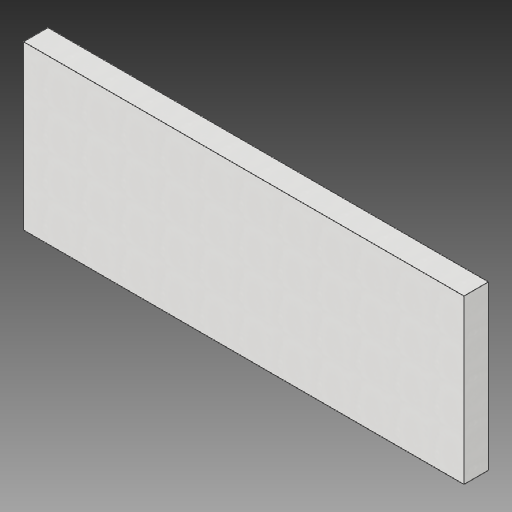
# Autodesk Inventor part: Перекрытие коридора
Saved by Autodesk Inventor 2019 (Build 230136000, 136)
## iProperties
Created: 2018-10-10
Part Number: Перекрытие коридора
Material: Гипсокартон
Document SubType Name: Modeling
Designer: Андреев Н.Л.
Density: 1.1 g/cm^3
Appearance: Гипсокартон — окрашенный — белый
Author: Андреев Н.Л.
Autodesk Inventor part; units mm, degrees
ref_plane "YZ Plane" through (0, 0, 0) normal (1, 0, 0) x (0, 1, 0)
ref_plane "XZ Plane" through (0, 0, 0) normal (0, 1, 0) x (-1, 0, 0)
ref_plane "XY Plane" through (0, 0, 0) normal (0, 0, 1) x (1, 0, 0)
sketch "Эскиз1" plane through (0, 0, 0) normal (0, 0, 1) x (1, 0, 0)
  line L0 (-1500, 2600) -> (-1500, -1200) construction
  line L1 (-1500, -1200) -> (-9900, -1200) construction
  line L2 (-9900, -1200) -> (-9900, 2600) construction
  line L3 (-9900, 2600) -> (-1500, 2600) construction
  line L4 (-1500, 3000) -> (-9900, 3000) construction
  line L5 (-9900, 3000) -> (-9900, 5000) construction
  line L6 (-9900, 5000) -> (-7000, 5000) construction
  line L7 (-7000, 5000) -> (-7000, 5400) construction
  line L8 (-7000, 5400) -> (-9900, 5400) construction
  line L9 (-9900, 5400) -> (-9900, 9200) construction
  line L10 (-9900, 9200) -> (-1500, 9200) construction
  line L11 (-1500, 9200) -> (-1500, 3000) construction
  line L12 (-10300, -200) -> (-10300, -1600) construction
  line L13 (-10300, -1600) -> (-1100, -1600) construction
  line L14 (-1100, -1600) -> (-1100, -200) construction
  line L15 (-1100, -200) -> (1100, -200) construction
  line L16 (1100, -200) -> (1100, -600) construction
  line L17 (1100, -600) -> (7500, -600) construction
  line L18 (7500, -600) -> (7500, 8600) construction
  line L19 (7500, 8600) -> (1100, 8600) construction
  line L20 (1100, 8600) -> (1100, 8200) construction
  line L21 (1100, 8200) -> (-1100, 8200) construction
  line L22 (-1100, 8200) -> (-1100, 9600) construction
  line L23 (-1100, 9600) -> (-10300, 9600) construction
  line L24 (-10300, 9600) -> (-10300, 8600) construction
  line L25 (-10300, 8600) -> (-18900, 8600) construction
  line L26 (-18900, 8600) -> (-18900, -600) construction
  line L27 (-18900, -600) -> (-12500, -600) construction
  line L28 (-12500, -600) -> (-12500, -200) construction
  line L29 (-12500, -200) -> (-10300, -200) construction
  line L30 (-1100, 7800) -> (1100, 7800) construction
  line L31 (1100, 7800) -> (1100, 200) construction
  line L32 (1100, 200) -> (-1100, 200) construction
  line L33 (-1100, 200) -> (-1100, 7800) construction
  line L34 (-18500, -200) -> (-18500, 8200) construction
  line L35 (-18500, 8200) -> (-12900, 8200) construction
  line L36 (-12900, 8200) -> (-12900, -200) construction
  line L37 (-12900, -200) -> (-18500, -200) construction
  line L38 (1500, -200) -> (1500, 8200) construction
  line L39 (1500, 8200) -> (7100, 8200) construction
  line L40 (7100, 8200) -> (7100, -200) construction
  line L41 (7100, -200) -> (1500, -200) construction
  line L42 (-10300, 200) -> (-12500, 200) construction
  line L43 (-12500, 200) -> (-12500, 8200) construction
  line L44 (-12500, 8200) -> (-10300, 8200) construction
  line L45 (-10300, 8200) -> (-10300, 200) construction
  line L46 (-6900, 3000) -> (-1500, 3000)
  line L47 (-1500, 3000) -> (-1500, 5000)
  line L48 (-1500, 5000) -> (-6900, 5000)
  line L49 (-6900, 5000) -> (-6900, 3000)
  point P0 (0, 0)
  dimension "d0" = 3000
  constraints: 8 end point, 2 parallel, 2 point on line, 1 collinear, 1 horizontal, 1 perpendicular
  measures "d0" distance between parallel lines of L49 L5
extrude "Выдавливание1" add sketch "Эскиз1" against normal blind 300
equation "\"d0\" = зДл"
equation "\"d1\" = зТолПерекрытия"
equation "\"зДл\" = 3000"
equation "\"пПодъем\" = 162.5"
equation "\"пХод\" = 296.8"
equation "\"пЭффШаг\" = 621.8"
equation "\"пСвес\" = 30.2"
equation "\"пОтступСтен\" = 5"
equation "\"пДиаг\" = 338.3733"
equation "\"пШирПроступи\" = 327"
equation "\"пТолПодступенка\" = 17.4"
equation "\"пГлубПаза\" = 12"
equation "\"пОтступОтСтен\" = 5"
equation "\"пТолПричала\" = 17.4"
equation "\"зТолПерекрытия\" = 300"
